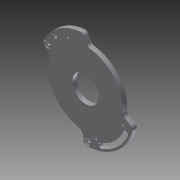
# Autodesk Inventor part: motor plate
Saved by Autodesk Inventor 2012 (Build 160160000, 160)
## iProperties
Created: 2012-01-30
Part Number: motor plate
Material: Default
Document SubType Name: Modeling
Designer: Antonella Wilby
Density: 1 g/cm^3
Author: Antonella Wilby
Autodesk Inventor part; units mm, degrees
ref_plane "YZ Plane" through (0, 0, 0) normal (1, 0, 0) x (0, 1, 0)
ref_plane "XZ Plane" through (0, 0, 0) normal (0, 1, 0) x (-1, 0, 0)
ref_plane "XY Plane" through (0, 0, 0) normal (0, 0, 1) x (1, 0, 0)
sketch "Sketch1" plane through (0, 0, 0) normal (0, 0, 1) x (1, 0, 0)
  circle A0 centre (0, 0) radius 53.975 construction
  line L0 (-138.9624, -14.2875) -> (-138.9624, 14.2875) construction
  circle A1 centre (0, 0) radius 19.05
  line L1 (-181.8914, 0) -> (118.6116, 0) projected
  line L2 (0, -111.81) -> (0, 105.5438) projected
  line L3 (-3.175, -62.217) -> (-3.175, -64.2153)
  arc A2 (-52.8351, 11.0342) -> (-10.795, -52.8845) centre (0, 0) ccw
  arc A3 (-52.8351, 11.0342) -> (-55.4238, 19.7166) centre (-62.1589, 12.9814) ccw
  arc A4 (-3.175, -62.217) -> (-10.795, -52.8845) centre (-12.7, -62.217) ccw
  arc A5 (53.9096, -2.6565) -> (6.1993, 53.6178) centre (0, 0) ccw
  line L4 (1.9382, 56.6066) -> (-2.1738, 64.8531)
  arc A6 (3.4886, -70.5576) -> (67.6849, -20.231) centre (0, 0) ccw
  arc A7 (-7.6764, 67.8434) -> (-60.7093, 31.2417) centre (0, 0) ccw
  arc A8 (1.9382, 56.6066) -> (6.1993, 53.6178) centre (6.8266, 59.0442) ccw
  arc A9 (-2.1738, 64.8531) -> (-7.6764, 67.8434) centre (-7.0623, 62.4156) ccw
  line L5 (57.0769, -8.4682) -> (64.7759, -12.9132)
  arc A10 (53.9096, -2.6565) -> (57.0769, -8.4682) centre (60.2519, -2.969) ccw
  arc A11 (67.6849, -20.231) -> (64.7759, -12.9132) centre (61.6009, -18.4125) ccw
  arc A12 (-3.175, -64.2153) -> (3.4886, -70.5576) centre (3.175, -64.2153) ccw
  line L6 (-55.4238, 19.7166) -> (-59.5532, 23.846)
  arc A13 (-60.7093, 31.2417) -> (-59.5532, 23.846) centre (-55.063, 28.3361) ccw
  point P0 (-3.175, -53.8815)
  point P1 (-50.8, 57.9383)
  point P2 (-3.175, -53.8815)
  point P3 (-3.175, -70.4964)
  point P4 (-67.8823, 0)
  point P5 (3.3007, 53.874)
  point P6 (53.975, 0)
  point P7 (-3.8272, 68.169)
  point P8 (53.5878, -6.4538)
  point P9 (68.9605, -15.3293)
  point P10 (-3.175, -70.5724)
  point P11 (-62.7098, 27.0026)
  dimension "d0" = 107.95
  dimension "d10" = 38.1
  dimension "d14" = 3.175
  dimension "d15" = 9.525
  dimension "d79" = 30
  dimension "d80" = 6.35
  dimension "d89" = 6.35
  dimension "d97" = 70.6437
  dimension "d98" = 6.35
  dimension "d108" = 45
  dimension "d109" = 5.4625
  dimension "d110" = 8.89
  constraints: 36 point on circle, 20 tangent, 14 centre point, 10 end point, 10 point on line, 4 coincident, 4 equal radius, 1 parallel
  measures "d0" diameter of A0
  measures "d10" diameter of A1
  measures "d14" distance between parallel lines of L2 L3
  measures "d15" radius of A3
  measures "d79" angle of L1 L5
  measures "d80" radius of A10
  measures "d89" radius of A12
  measures "d97" radius of A6
  measures "d98" radius of A13
  measures "d108" angle of L6 L1
  measures "d109" radius of A9
  measures "d110" distance of L5.start L5.end
extrude "Base" add sketch "Sketch1" along normal mid plane 6.35 contours L1 A5 A10 L5 A11 A6 A12 L2 A1 | A1 L2 L4 A8 A5 L1 | A1 L1 A2 A3 L6 A13 A7 A9 L4 L2 | L2 A12 L3 A4 A2 L1 A1
sketch "Sketch5" plane through (0, 0, -3.175) normal (0, 0, -1) x (-1, 0, 0)
  circle A0 centre (0, 0) radius 19.05 projected
  arc A1 (60.7093, 31.2417) -> (7.6764, 67.8434) centre (0, 0) ccw projected
  circle A2 centre (0, 0) radius 53.975 construction
  line L0 (-53.2759, -12.7) -> (-58.4475, -17.8716) construction
  line L1 (-9.2461, -53.9826) -> (-14.6103, -59.3468) construction
  line L2 (91.9487, 0) -> (-94.6008, 0) projected
  line L3 (0, -99.577) -> (0, 103.505) projected
  arc A3 (-53.2759, -12.7) -> (-9.2461, -53.9826) centre (0, 0) ccw construction
  arc A4 (28.575, 46.7235) -> (-28.575, 46.7235) centre (0, 0) ccw construction
  arc A5 (-58.4475, -17.8716) -> (-14.6103, -59.3468) centre (0, 0) ccw construction
  arc A6 (28.575, 54.0275) -> (-28.575, 54.0275) centre (0, 0) ccw construction
  line L4 (-28.575, 46.7235) -> (-28.575, 54.0275) construction
  line L5 (28.575, 46.7235) -> (28.575, 54.0275) construction
  point P0 (40.1638, 60.9879)
  point P1 (-25.4, 51.9032)
  point P2 (25.4, 51.9032)
  point P3 (-54.2025, -18.1167)
  point P4 (-14.9213, -55.1677)
  dimension "d55" = 107.95
  dimension "d56" = 60.325
  dimension "d57" = 6.35
  dimension "d58" = 0.7937
  dimension "d59" = 57.15
  dimension "d60" = 6.35
  dimension "d61" = 0.7937
  dimension "d65" = 3.175
  dimension "d66" = 3.175
  dimension "d67" = 57.785
  dimension "d82" = 45
  dimension "d83" = 12.7
  dimension "d84" = 3.175
  dimension "d85" = 3.175
  dimension "d87" = 57.15
  dimension "d88" = 57.15
  constraints: 8 end point, 8 point on circle, 5 centre point, 3 parallel, 1 coincident, 1 horizontal alignment, 2 other
  measures "d55" diameter of A2
  measures "d56" distance between parallel lines of L1 L0
  measures "d57" radial gap between concentric circles of A3 A5
  measures "d58" radial gap between concentric circles of A2 A3
  measures "d59" distance between parallel lines of L5 L4
  measures "d60" radial gap between concentric circles of A6 A4
  measures "d61" radial gap between concentric circles of A4 A2
  measures "d65" distance from line of point (-25.4, 51.903) L4
  measures "d66" distance from line of L5 point (25.4, 51.903)
  measures "d67" distance of point (-25.4, 51.903) A0.centre
  measures "d82" angle of L2 L0
  measures "d83" distance from line of L2 L0.start
  measures "d84" distance from line of L0 point (-54.202, -18.117)
  measures "d85" distance from line of point (-14.921, -55.168) L1
  measures "d87" distance of A2.centre point (-54.202, -18.117)
  measures "d88" distance of A2.centre point (-14.921, -55.168)
hole "Motor Stay Holes" at (25.4, 51.9032, -3.175) at (-25.4, 51.9032, -3.175) at (14.9213, -55.1677, -3.175) at (54.2025, -18.1167, -3.175) direction (0, 0, 1) diameter 3.175 end through all
sketch "Sketch6" plane through (0, 0, 3.175) normal (0, 0, 1) x (1, 0, 0)
  arc A0 (-3.175, -64.2153) -> (3.4886, -70.5576) centre (3.175, -64.2153) ccw projected
  arc A1 (-60.7093, 31.2417) -> (-59.5532, 23.846) centre (-55.063, 28.3361) ccw projected
  constraints: 2 coincident
hole "Standoff Holes to front plate" at (3.175, -64.2153, 3.175) at (-55.063, 28.3361, 3.175) direction (0, 0, -1) diameter 5.1054 end through all counterbore diameter 9.779 counterbore depth 1.5875 clearance for "Flat Head Machine Screw (82)" size "#10" standard "Ansi Unified Screw Threads"
sketch "Sketch8" plane through (0, 0, -3.175) normal (0, 0, -1) x (-1, 0, 0)
  arc A0 (59.5532, 23.846) -> (60.7093, 31.2417) centre (55.063, 28.3361) ccw projected
  arc A1 (60.7093, 31.2417) -> (7.6764, 67.8434) centre (0, 0) ccw projected
  circle A2 centre (0, 0) radius 61.9263 construction
  arc A3 (10.795, -52.8845) -> (52.8351, 11.0342) centre (0, 0) ccw projected
  line L0 (0, 0) -> (43.7885, 43.7885) construction
  line L1 (94.4751, 0) -> (-104.0422, 0) projected
  line L2 (0, -111.81) -> (0, 105.5438) projected
  dimension "d119" = 45
  constraints: 2 end point, 2 point on circle, 1 centre point, 1 coincident
  measures "d119" angle of L0 L1
hole "Standoff Holes to back plate" at (-43.7885, 43.7885, -3.175) direction (0, 0, 1) diameter 5.1054 end through all counterbore diameter 9.779 counterbore depth 1.5875 clearance for "Flat Head Machine Screw (82)" size "#10" standard "Ansi Unified Screw Threads"
sketch "Sketch7" plane through (0, 0, 3.175) normal (0, 0, 1) x (1, 0, 0)
  arc A0 (3.4886, -70.5576) -> (67.6849, -20.231) centre (0, 0) ccw projected
  arc A1 (20.7648, -57.0509) -> (23.0757, -63.3999) centre (21.9203, -60.2254) ccw
  arc A2 (61.1475, -28.5135) -> (55.0241, -25.6581) centre (58.0858, -27.0858) ccw
  arc A3 (23.0757, -63.3999) -> (61.1475, -28.5135) centre (0, 0) ccw
  arc A4 (20.7648, -57.0509) -> (55.0241, -25.6581) centre (0, 0) ccw
  line L0 (58.0858, -27.0858) -> (0, 0) construction
  line L1 (0, 0) -> (21.9203, -60.2254) construction
  line L2 (-88.8322, 0) -> (103.1018, 0) projected
  line L3 (0, -110.4869) -> (0, 97.6056) projected
  dimension "d102" = 3.175
  dimension "d103" = 6.7564
  dimension "d104" = 25
  dimension "d105" = 20
  constraints: 8 point on circle, 4 centre point, 4 end point, 4 tangent
  measures "d102" radial gap between concentric circles of A3 A0
  measures "d103" radial gap between concentric circles of A4 A3
  measures "d104" angle of L2 L0
  measures "d105" angle of L3 L1
extrude "Tensioning Slot" cut sketch "Sketch7" against normal through all
body "Solid1"
